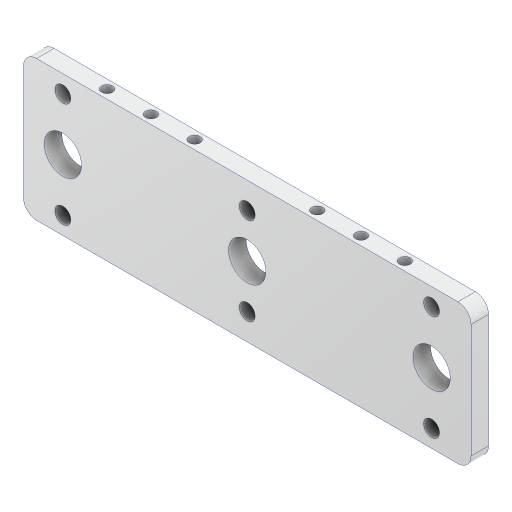
# Autodesk Inventor part: 스프링블럭2
Saved by Autodesk Inventor 2023.2 (Build 272271000, 271)
## iProperties
Created: 2022-12-27
Part Number: 스프링블럭2
Material: 알루미늄 6061
Document SubType Name: Modeling
Designer: BAEK
Density: 2.7 g/cm^3
Appearance: 알루미늄 - 평지
Mass: 32.7388 g
Surface Area: 77.0761 cm^2
Volume: 12.1255 cm^3
Author: BAEK
Autodesk Inventor part; units mm, degrees
ref_plane "YZ Plane" through (0, 0, 0) normal (1, 0, 0) x (0, 1, 0)
ref_plane "XZ Plane" through (0, 0, 0) normal (0, 1, 0) x (-1, 0, 0)
ref_plane "XY Plane" through (0, 0, 0) normal (0, 0, 1) x (1, 0, 0)
sketch "스케치1" plane through (0, 0, 0) normal (0, 0, 1) x (1, 0, 0)
  line L0 (-48.1, 15) -> (48.1, 15)
  line L1 (48.1, 15) -> (48.1, -15)
  line L2 (48.1, -15) -> (-48.1, -15)
  line L3 (-48.1, -15) -> (-48.1, 15)
  line L4 (-48.1, 15) -> (48.1, -15) construction
  line L5 (48.1, 15) -> (-48.1, -15) construction
  point P0 (0, 0)
  dimension "d0" = 96.2
  dimension "d1" = 30
  constraints: 12 end point, 2 midpoint, 2 parallel, 1 horizontal, 1 perpendicular
  measures "d0" distance of L1.end L2.end
  measures "d1" distance of L0.end L1.end
extrude "돌출1" add sketch "스케치1" along normal blind 4
sketch "스케치2" plane through (0, 0, 4) normal (0, 0, 1) x (1, 0, 0)
  circle A0 centre (42.1, 0) radius 4.25
  circle A1 centre (-42.1, 0) radius 4.25
  arc A2 (-46.1, 15) -> (-48.1, 13) centre (-46.1, 13) ccw
  line L0 (-48.1, 13) -> (-48.1, -13)
  arc A3 (-48.1, -13) -> (-46.1, -15) centre (-46.1, -13) ccw
  line L1 (-46.1, -15) -> (46.1, -15)
  arc A4 (46.1, -15) -> (48.1, -13) centre (46.1, -13) ccw
  line L2 (48.1, -13) -> (48.1, 13)
  arc A5 (48.1, 13) -> (46.1, 15) centre (46.1, 13) ccw
  line L3 (46.1, 15) -> (-46.1, 15)
  circle A6 centre (12, 0) radius 1.35
  circle A7 centre (0, 12) radius 1.35
  circle A8 centre (-12, 0) radius 1.35
  circle A9 centre (42.1, -12) radius 1.8
  circle A10 centre (-42.1, -12) radius 1.8
  circle A11 centre (42.1, 12) radius 1.8
  circle A12 centre (-42.1, 12) radius 1.8
  line L4 (-48.1, -15) -> (48.1, -15) projected
  line L5 (48.1, -15) -> (48.1, 15) projected
  line L6 (48.1, 15) -> (-48.1, 15) projected
  line L7 (-48.1, 15) -> (-48.1, -15) projected
  point P0 (0, 0)
  point P1 (0, 0)
  point P2 (48.1, -13)
  point P3 (-48.1, 13)
  dimension "d4" = 8.5
  dimension "d5" = 92.2
  dimension "d6" = 26
  dimension "d7" = 8.5
  dimension "d8" = 15
  dimension "d9" = 15
  dimension "d10" = 6
  dimension "d11" = 6
  dimension "d12" = 12
  dimension "d13" = 12
  dimension "d14" = 3.6
  dimension "d15" = 3.6
  dimension "d16" = 3.6
  dimension "d17" = 3.6
  dimension "d18" = 12
  dimension "d19" = 12
  dimension "d20" = 2.7
  dimension "d21" = 2.7
  dimension "d22" = 2.7
  dimension "d25" = 12
  dimension "d26" = 24
  constraints: 13 centre point, 8 end point, 8 point on circle, 1 horizontal alignment
  measures "d4" diameter of A1
  measures "d5" distance of L3.start L3.end
  measures "d6" distance of L2.start L2.end
  measures "d7" diameter of A0
  measures "d8" distance from line of L3 A1.centre
  measures "d9" distance from line of L3 A0.centre
  measures "d10" distance from line of L0 A1.centre
  measures "d11" distance from line of L2 A0.centre
  measures "d12" distance of A12.centre A1.centre
  measures "d13" distance of A1.centre A10.centre
  measures "d14" diameter of A10
  measures "d15" diameter of A12
  measures "d16" diameter of A11
  measures "d17" diameter of A9
  measures "d18" distance of A0.centre A9.centre
  measures "d19" distance of A0.centre A11.centre
  measures "d20" diameter of A8
  measures "d21" diameter of A7
  measures "d22" diameter of A6
  measures "d25" horizontal distance of A7.centre A6.centre
  measures "d26" distance of A8.centre A6.centre
extrude "돌출2" cut sketch "스케치2" against normal blind 4 contours A0 | A1 | A2 L7 L6 | L6 L5 A5 | A3 L4 L7 | L5 L4 A4 | A6 | A7 | A8 | A9 | A10 | A11 | A12
sketch "스케치3" plane through (0, 0, 4) normal (0, 0, 1) x (1, 0, 0)
  circle A0 centre (-12, 0) radius 1.35 projected
  circle A1 centre (42.1, 0) radius 4.25 projected
  circle A2 centre (-42.1, -12) radius 1.8 projected
  circle A3 centre (42.1, 12) radius 1.8 projected
  circle A4 centre (0, 12) radius 1.35 projected
  circle A5 centre (-42.1, 0) radius 4.25 projected
  circle A6 centre (-42.1, 12) radius 1.8 projected
  circle A7 centre (42.1, -12) radius 1.8 projected
  circle A8 centre (12, 0) radius 1.35 projected
  arc A9 (46.1, -15) -> (48.1, -13) centre (46.1, -13) ccw projected
  line L0 (48.1, -13) -> (48.1, 13) projected
  arc A10 (48.1, 13) -> (46.1, 15) centre (46.1, 13) ccw projected
  line L1 (46.1, 15) -> (-46.1, 15) projected
  arc A11 (-46.1, 15) -> (-48.1, 13) centre (-46.1, 13) ccw projected
  line L2 (-48.1, 13) -> (-48.1, -13) projected
  arc A12 (-48.1, -13) -> (-46.1, -15) centre (-46.1, -13) ccw projected
  line L3 (-46.1, -15) -> (46.1, -15) projected
  line L4 (-48.1, 13) -> (-48.1, -13) projected
  line L5 (-48.1, 13) -> (-48.1, 16)
  arc A13 (48.1, 13) -> (46.1, 15) centre (46.1, 13) ccw projected
  line L6 (48.1, 13) -> (48.1, 16)
  line L7 (48.1, 16) -> (-48.1, 16)
  line L8 (48.1, -13) -> (48.1, 13) projected
  line L9 (48.1, -13) -> (48.1, -16)
  line L10 (-48.1, -13) -> (-48.1, -16)
  line L11 (-48.1, -16) -> (48.1, -16)
  point P0 (0, 0)
  dimension "d29" = 3
  dimension "d30" = 3
  dimension "d31" = 3
  dimension "d32" = 3
  constraints: 12 end point, 2 point on line, 2 tangent, 1 collinear, 1 vertical
  measures "d29" distance of L2.start L5.end
  measures "d30" distance of L0.end L6.end
  measures "d31" distance of L0.start L9.end
  measures "d32" distance of L2.end L10.end
extrude "돌출3" add sketch "스케치3" against normal blind 4 contours A9 L9 L11 L10 A12 L3 | A10 L1 A11 L5 L7 L6
fillet "모깎기1" radius 3 4 edges at (-48.1, -16, 2) (48.1, -16, 2) (48.1, 16, 2) (-48.1, 16, 2)
sketch "스케치4" plane through (0, 0, 4) normal (0, 0, 1) x (1, 0, 0)
  arc A0 (-45.1, 16) -> (-48.1, 13) centre (-45.1, 13) ccw projected
  line L0 (-48.1, 13) -> (-48.1, -13) projected
  arc A1 (-48.1, -13) -> (-45.1, -16) centre (-45.1, -13) ccw projected
  line L1 (-45.1, -16) -> (45.1, -16) projected
  arc A2 (45.1, -16) -> (48.1, -13) centre (45.1, -13) ccw projected
  line L2 (48.1, -13) -> (48.1, 13) projected
  arc A3 (48.1, 13) -> (45.1, 16) centre (45.1, 13) ccw projected
  line L3 (45.1, 16) -> (-45.1, 16) projected
  circle A4 centre (-12, 0) radius 1.35 projected
  circle A5 centre (42.1, 0) radius 4.25 projected
  circle A6 centre (-42.1, -12) radius 1.8 projected
  circle A7 centre (42.1, 12) radius 1.8 projected
  circle A8 centre (0, 12) radius 1.35 projected
  circle A9 centre (-42.1, 0) radius 4.25 projected
  circle A10 centre (-42.1, 12) radius 1.8 projected
  circle A11 centre (42.1, -12) radius 1.8 projected
  circle A12 centre (12, 0) radius 1.35 projected
  line L4 (45.1, 16) -> (-45.1, 16) projected
  line L5 (-45.1, 16) -> (-51.1, 16)
  arc A13 (-45.1, 16) -> (-48.1, 13) centre (-45.1, 13) ccw projected
  line L6 (-51.1, 16) -> (-51.1, -16)
  line L7 (-45.1, -16) -> (45.1, -16) projected
  line L8 (-51.1, -16) -> (-45.1, -16)
  line L9 (45.1, 16) -> (51.1, 16)
  line L10 (51.1, 16) -> (51.1, -16)
  line L11 (51.1, -16) -> (45.1, -16)
  point P0 (0, 0)
  dimension "d36" = 6
  dimension "d37" = 6
  constraints: 12 end point, 2 perpendicular, 1 horizontal, 1 point on line, 1 tangent, 1 vertical
  measures "d36" distance of L3.end L5.end
  measures "d37" distance of L3.start L9.end
extrude "돌출4" add sketch "스케치4" against normal blind 4 contours A0 L0 A1 L8 L6 L5 | L9 L10 L11 A2 L2 A3
fillet "모깎기2" radius 3 4 edges at (-51.1, -16, 2) (-51.1, 16, 2) (51.1, 16, 2) (51.1, -16, 2)
sketch "스케치5" plane through (0, 0, 4) normal (0, 0, 1) x (1, 0, 0)
  circle A0 centre (0, 0) radius 4.25
  dimension "d41" = 8.5
  constraints: 1 centre point, 1 coincident
  measures "d41" diameter of A0
extrude "돌출5" cut sketch "스케치5" against normal blind 4
sketch "스케치6" plane through (0, 0, 4) normal (0, 0, 1) x (1, 0, 0)
  line L0 (0, 0) -> (0, 10)
  circle A0 centre (0, 0) radius 4.25 projected
  line L1 (0, 0) -> (0, -10)
  circle A1 centre (0, 10) radius 1.8
  circle A2 centre (0, -10) radius 1.8
  circle A3 centre (0, 0) radius 4.25 projected
  arc A4 (48.1, -16) -> (51.1, -13) centre (48.1, -13) ccw projected
  line L2 (51.1, -13) -> (51.1, 13) projected
  arc A5 (51.1, 13) -> (48.1, 16) centre (48.1, 13) ccw projected
  line L3 (48.1, 16) -> (-48.1, 16) projected
  arc A6 (-48.1, 16) -> (-51.1, 13) centre (-48.1, 13) ccw projected
  line L4 (-51.1, 13) -> (-51.1, -13) projected
  arc A7 (-51.1, -13) -> (-48.1, -16) centre (-48.1, -13) ccw projected
  line L5 (-48.1, -16) -> (48.1, -16) projected
  circle A8 centre (-12, 0) radius 1.35 projected
  circle A9 centre (42.1, 0) radius 4.25 projected
  circle A10 centre (-42.1, -12) radius 1.8 projected
  circle A11 centre (42.1, 12) radius 1.8 projected
  circle A12 centre (0, 12) radius 1.35 projected
  circle A13 centre (-42.1, 0) radius 4.25 projected
  circle A14 centre (-42.1, 12) radius 1.8 projected
  circle A15 centre (42.1, -12) radius 1.8 projected
  circle A16 centre (12, 0) radius 1.35 projected
  dimension "d44" = 10
  dimension "d45" = 10
  dimension "d46" = 3.6
  dimension "d47" = 3.6
  constraints: 4 end point, 2 centre point, 2 coincident, 2 vertical
  measures "d44" distance of L0.start L0.end
  measures "d45" distance of L1.start L1.end
  measures "d46" diameter of A1
  measures "d47" diameter of A2
extrude "돌출6" add sketch "스케치6" against normal blind 4 contours A12 A1 | A1 A12 | A8 | A16 picked at (0.3966, 12.2209) picked at (0.1959, 11.4027)
extrude "돌출7" cut sketch "스케치6" against normal blind 4 contours A1 A12 | A2 | A1 A12 picked at (-0.1974, 9.0374) picked at (0.1959, 11.4027)
sketch "스케치8" plane through (-48.1, -16, 4) normal (0, -1, 0) x (1, 0, 0)
  line L0 (96.2, 0) -> (96.2, -4) projected
  line L1 (0, 0) -> (96.2, 0) projected
  line L2 (0, -4) -> (0, 0) projected
  line L3 (96.2, -4) -> (0, -4) projected
  line L4 (96.2, -4) -> (96.2, 0) projected
  line L5 (96.2, -2) -> (0, -2) construction
  line L6 (0, -4) -> (0, 0) projected
  line L7 (48.1, -4) -> (48.1, 0) construction
  circle A0 centre (34.1, -2) radius 1.25
  circle A1 centre (24.1, -2) radius 1.25
  circle A2 centre (14.1, -2) radius 1.25
  circle A3 centre (62.1, -2) radius 1.25
  circle A4 centre (72.1, -2) radius 1.25
  circle A5 centre (82.1, -2) radius 1.25
  point P0 (48.1, -2)
  dimension "d53" = 2.5
  dimension "d54" = 2.5
  dimension "d55" = 2.5
  dimension "d56" = 2.5
  dimension "d57" = 2.5
  dimension "d58" = 2.5
  dimension "d59" = 14
  dimension "d60" = 10
  dimension "d61" = 10
  dimension "d63" = 10
  dimension "d64" = 10
  dimension "d67" = 14
  constraints: 6 centre point, 3 midpoint, 2 end point, 10 other
  measures "d53" diameter of A0
  measures "d54" diameter of A1
  measures "d55" diameter of A2
  measures "d56" diameter of A3
  measures "d57" diameter of A4
  measures "d58" diameter of A5
  measures "d59" distance of point (48.1, -2) A0.centre
  measures "d60" distance of A1.centre A2.centre
  measures "d61" distance of A1.centre A0.centre
  measures "d63" distance of A4.centre A3.centre
  measures "d64" distance of A5.centre A4.centre
  measures "d67" distance of point (48.1, -2) A3.centre
extrude "돌출8" cut sketch "스케치8" against normal blind 4 contours A0 | A1 | A2 | A3 | A4 | A5
mirror "미러1" about plane through (0, 0, 0) normal (0, 1, 0) of "돌출8"
